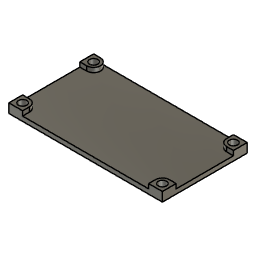
StepUpDrzak v2 (Autodesk Fusion 360 design; units mm, degrees)
Autodesk Fusion 360 part; units mm, degrees
sketch "Sketch1" plane through (0, 0, 0) normal (0, 0, 1) x (1, 0, 0)
  circle A0 centre (0, 0) radius 1.8
  circle A1 centre (61, 0) radius 1.8
  circle A2 centre (0, 31) radius 1.8
  circle A3 centre (61, 31) radius 1.8
  line L0 (-3, 34) -> (64, 34)
  line L1 (64, 34) -> (64, -3)
  line L2 (64, -3) -> (-3, -3)
  line L3 (-3, -3) -> (-3, 34)
  dimension "d3" = 61
  dimension "d4" = 31
  dimension "d5" = 3.6
  dimension "d6" = 3
  dimension "d7" = 3
  dimension "d8" = 3
  dimension "d9" = 3
  constraint coincident A0.centre origin
  constraint horizontal L0
  constraint vertical L1
  constraint horizontal L2
  constraint vertical L3
  measures "d5" diameter of A0
  measures "d6" horizontal distance of A0.centre L2.end
  measures "d7" vertical distance of A0.centre L2.end
  measures "d8" horizontal distance of A3.centre L0.end
  measures "d9" vertical distance of A3.centre L0.end
extrude "Extrude1" add sketch "Sketch1" along normal blind 2
sketch "Sketch2" plane through (0, 0, 2) normal (0, 0, 1) x (-1, 0, 0)
  circle A0 centre (0, 0) radius 1.8
  circle A1 centre (-61, 0) radius 1.8
  circle A2 centre (-61, -31) radius 1.8
  circle A3 centre (0, -31) radius 1.8
  line L0 (3, 3) -> (-64, 3)
  line L1 (-64, 3) -> (-64, -34)
  line L2 (-64, -34) -> (3, -34)
  line L3 (3, -34) -> (3, 3)
  circle A4 centre (0, -31) radius 3
  line L4 (-3, -31) -> (-3, -34)
  line L5 (0, -28) -> (3, -28)
  circle A5 centre (-61, -31) radius 3
  line L6 (-61, -28) -> (-64, -28)
  line L7 (-58, -31) -> (-58, -34)
  circle A6 centre (-61, 0) radius 3
  line L8 (-58, 0) -> (-58, 3)
  line L9 (-61, -3) -> (-64, -3)
  circle A7 centre (0, 0) radius 3
  line L10 (-3, 0) -> (-3, 3)
  line L11 (0, -3) -> (3, -3)
  constraint concentric A3 A4
  constraint tangent L2 A4
  constraint coincident A4 L4.start
  constraint coincident L2 L4.end
  constraint tangent A4 L4
  constraint perpendicular L2 L4
  constraint coincident A4 L5.start
  constraint coincident L3 L5.end
  constraint tangent A4 L5
  constraint perpendicular L3 L5
  constraint concentric A2 A5
  constraint tangent L2 A5
  constraint coincident A5 L6.start
  constraint coincident L1 L6.end
  constraint tangent A5 L6
  constraint perpendicular L1 L6
  constraint coincident A5 L7.start
  constraint coincident L2 L7.end
  constraint tangent A5 L7
  constraint perpendicular L2 L7
  constraint concentric A1 A6
  constraint tangent L1 A6
  constraint coincident A6 L8.start
  constraint coincident L0 L8.end
  constraint tangent A6 L8
  constraint perpendicular L0 L8
  constraint coincident A6 L9.start
  constraint coincident L1 L9.end
  constraint tangent A6 L9
  constraint perpendicular L1 L9
  constraint coincident A0.centre A7.centre
  constraint tangent L0 A7
  constraint coincident A7 L10.start
  constraint coincident L0 L10.end
  constraint tangent A7 L10
  constraint perpendicular L0 L10
  constraint coincident A7 L11.start
  constraint coincident L3 L11.end
  constraint tangent A7 L11
  constraint perpendicular L3 L11
extrude "Extrude2" add sketch "Sketch2" along normal blind 2 contours L0 A7 L10 | L0 A6 L8 | L0 L3 A7 | A7 | L0 L1 A6 | A6 | L3 A7 L11 | L1 A6 L9 | L3 A4 L5 | L1 A5 L6 | A4 | L2 L3 A4 | L1 L2 A5 | A5 | L2 A5 L7
equation "d7 = d6"
equation "d8 = d6"
equation "d9 = d6"
